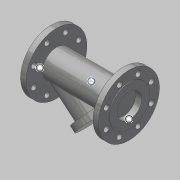
# Autodesk Inventor part: STRAINER Y-TYPE FLANGED GGG50 DN80
Saved by Autodesk Inventor 2017 (Build 210142000, 142)
## iProperties
Category: Piping Part
Company: Pocket Brewery Belgium
Created: 2012-12-20
Part Number: STRAINER Y-TYPE FLANGED GGG50 DN80
Material: GGG50
Document SubType Name: Modeling
Designer: Marc Crauwels
Density: 7.85 g/cm^3
Mass: 658107 g
Surface Area: 21375.3 cm^2
Volume: 83622.3 cm^3
Appearance: Steel
Catalog Web Link: http://www.pocketbrewery.com
Author: Marc Crauwels
Title: Carbon Steel Globe Valve PN16
Comments: iPart CS GlbVlvPN16
Autodesk Inventor part; units mm, degrees
ref_plane "YZ Plane" through (0, 0, 0) normal (1, 0, 0) x (0, 1, 0)
ref_plane "XZ Plane" through (0, 0, 0) normal (0, 1, 0) x (-1, 0, 0)
ref_plane "XY Plane" through (0, 0, 0) normal (0, 0, 1) x (1, 0, 0)
sketch "Sketch1" plane through (0, 0, 0) normal (1, 0, 0) x (0, 1, 0)
  line L0 (110, 40) -> (128, 40)
  line L1 (128, 40) -> (128, 100)
  line L2 (128, 100) -> (110, 100)
  line L3 (110, 100) -> (110, 40)
  line L4 (128, 40) -> (130, 40)
  line L5 (130, 40) -> (130, 66)
  line L6 (130, 66) -> (128, 66)
  line L7 (128, 66) -> (128, 40)
  line L8 (-130, 0) -> (130, 0) construction
  line L9 (130, 0) -> (110, 0) construction
  line L10 (0, 0) -> (0, 218.263545) construction
  line L11 (-130, 0) -> (-110, 0) construction
  line L12 (0, 0) -> (-5.078912, 0)
  dimension "Lenght" = 260
  dimension "DN" = 80
  dimension "FlgDia" = 200
  dimension "FlgThck" = 20
  dimension "GsktFace" = 132
  dimension "Face" = 2
  constraints: 26 end point, 5 point on line, 4 parallel, 3 horizontal, 3 perpendicular, 2 coincident, 2 collinear, 1 midpoint
  measures "Lenght" distance of L8.start L8.end
  measures "DN" diameter of L0 L8
  measures "FlgDia" diameter of L2 L8
  measures "FlgThck" distance between parallel lines of L3 L5
  measures "GsktFace" diameter of L5.end L8
  measures "Face" distance of L5.end L6.end
revolve "Revolution1" add sketch "Sketch1" angle 360 about axis through (0, -130, 0) along (0, 1, 0)
sketch "Sketch5" plane through (0, 128, 0) normal (0, 1, 0) x (1, 0, 0)
  line L0 (0, 0) -> (-30.614675, 73.910363)
  line L1 (0, 0) -> (0, 224.469147) construction
  circle A0 centre (-30.614675, 73.910363) radius 9
  point P0 (0, 0)
  dimension "d16" = 80
  dimension "d17" = 22.5
  dimension "d18" = 18
  constraints: 4 end point, 2 coincident, 1 centre point, 1 vertical
  measures "d16" distance of L0.start L0.end
  measures "d17" angle of L1 L0
  measures "d18" diameter of A0
extrude "Extrusion2" cut sketch "Sketch5" against normal through all
pattern_circular "Circular Pattern1" count 8 over 360 about axis through (0, 129, 0) along (0, 1, 0) of "Extrusion2"
sketch "Sketch14" plane through (0, 110, 0) normal (0, -1, 0) x (-1, 0, 0)
  circle A0 centre (0, 0) radius 40 projected
  circle A1 centre (0, 0) radius 46
  dimension "d54" = 6
  constraints: 1 centre point
  measures "d54" radial gap between concentric circles of A1 A0
pattern_circular "Circular Pattern2" count 2 over 360 about axis through (-10, 0, 0) along (1, 0, 0) of "Revolution1", "Extrusion2", "Circular Pattern1"
extrude "Extrusion5" add sketch "Sketch14" along normal up to surface (220 mm away) contours A0 | A1
sketch "Sketch21 outline for Revolution5" plane through (0, 0, 0) normal (1, 0, 0) x (0, 1, 0)
  line L0 (110, 6.20619) -> (-15.612795, -99.146103)
  line L1 (110, -46) -> (110, 6.20619)
  line L2 (10.091642, -129.79381) -> (110, -46)
  line L3 (-15.612795, -99.146103) -> (10.091642, -129.79381)
revolve "Revolution5" add sketch "Sketch21 outline for Revolution5" angle 360 about axis through (0, -15.612795, -99.146103) along (0, 0.7661927, 0.6426109)
fillet "Fillet2" [suppressed]
sketch "Sketch22" plane through (0, -15.612795, -99.146103) normal (0, -0.7661927, -0.6426109) x (-1, 0, 0)
  circle A0 centre (0, 0) radius 40 projected
  circle A1 centre (0, 0) radius 55
  point P0 (0, -65.932064)
  dimension "d86" = 15
  constraints: 1 centre point
  measures "d86" radial gap between concentric circles of A0 A1
extrude "Extrusion8" add sketch "Sketch22" against normal blind 20 contours A0 | A1
sketch "Sketch21" plane through (0, 0, 0) normal (1, 0, 0) x (0, 1, 0)
  line L0 (-15.612795, -99.146103) -> (110, 6.20619)
  line L1 (0.204486, 6.20619) -> (71.258352, 6.20619) construction
  line L2 (-15.612795, -99.146103) -> (10.091642, -129.79381)
  line L3 (10.091642, -129.79381) -> (110, -46)
  line L4 (110, -46) -> (110, 6.20619)
  line L5 (110, -46) -> (-110.232314, -46)
  line L6 (-15.612795, -99.146103) -> (-41.317232, -68.498397) construction
  line L7 (-110, 100) -> (-110, -100)
  line L8 (-41.317232, -68.498397) -> (47.753937, 6.20619) construction
  line L9 (110, -46) -> (-110, -46)
  line L10 (-110, 100) -> (-110, -100)
  dimension "d79" = 40
  dimension "oH" = 136
  dimension "d89" = 20
  constraints: 16 end point, 5 perpendicular, 2 collinear, 2 point on line, 1 horizontal, 1 vertical, 3 other
  measures "d79" distance of L0.start L2.end
  measures "oH" vertical distance of L1.end L2.end
  measures "d89" distance from line of L10.end L8
equation "\"d16\" = 0.5 * KDia"
equation "\"KDia\" = 160"
body "Solid1"
